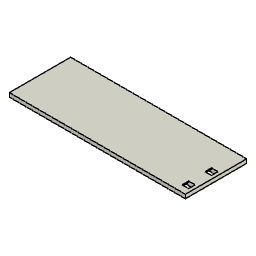
sorted_smarties_top_panel (Autodesk Fusion 360 design; units mm, degrees)
Autodesk Fusion 360 part; units mm, degrees
sketch "Sorted Smarties Top" plane through (0, 0, 0) normal (0, 0, 1) x (1, 0, 0)
  line L0 (0, 0) -> (-270, 0)
  line L1 (-270, 0) -> (-270, 94)
  line L2 (-270, 94) -> (0, 94)
  line L3 (0, 94) -> (0, 0)
  dimension "d2" = 270
  dimension "d3" = 94
  constraint horizontal L0
  constraint vertical L1
  constraint horizontal L2
  constraint vertical L3
  constraint coincident L0.start L3.end
  measures "d2" distance of L0.start L0.end
  measures "d3" distance of L0.start L2.end
extrude "Extrude1" add sketch "Sorted Smarties Top" along normal blind 6
sketch "Sketch2" plane through (0, 0, 0) normal (0, 0, -1) x (1, 0, 0)
  line L0 (-270, -94) -> (0, -94)
  line L1 (0, -94) -> (0, 0)
  line L2 (0, 0) -> (-270, 0)
  line L3 (-270, 0) -> (-270, -94)
  line L4 (-5, -10) -> (-265, -10)
  line L5 (-265, -10) -> (-265, -20)
  line L6 (-265, -20) -> (-5, -20)
  line L7 (-5, -20) -> (-5, -10)
  line L8 (-5, -45) -> (-265, -45)
  line L9 (-265, -45) -> (-265, -55)
  line L10 (-265, -55) -> (-5, -55)
  line L11 (-5, -55) -> (-5, -45)
  dimension "d6" = 10
  dimension "d7" = 10
  dimension "d8" = 10
  dimension "d9" = 25
  dimension "d10" = 5
  dimension "d11" = 5
  dimension "d12" = 5
  dimension "d13" = 5
  constraint horizontal L4
  constraint vertical L5
  constraint horizontal L6
  constraint vertical L7
  constraint horizontal L8
  constraint vertical L9
  constraint horizontal L10
  constraint vertical L11
  measures "d6" distance of L2 L4
  measures "d7" distance of L4.start L6.end
  measures "d8" distance of L8.start L10.end
  measures "d9" distance of L6 L8
  measures "d10" distance of L3 L5
  measures "d11" distance of L1 L7
  measures "d12" distance of L1 L11
  measures "d13" distance of L3 L9
extrude "Extrude2" cut sketch "Sketch2" against normal blind 4 contours L4 L5 L6 L7 | L8 L9 L10 L11
sketch "Sketch3" plane through (0, 0, 4) normal (0, 0, -1) x (1, 0, 0)
  line L0 (-5, -20) -> (-5, -10)
  line L1 (-5, -10) -> (-265, -10)
  line L2 (-265, -10) -> (-265, -20)
  line L3 (-265, -20) -> (-5, -20)
  line L4 (-5, -10) -> (-15, -10)
  line L5 (-15, -10) -> (-15, -20)
  line L6 (-15, -20) -> (-5, -20)
  line L7 (-5, -20) -> (-5, -10)
  line L8 (-5, -45) -> (-15, -45)
  line L9 (-15, -45) -> (-15, -55)
  line L10 (-15, -55) -> (-5, -55)
  line L11 (-5, -55) -> (-5, -45)
  constraint horizontal L4
  constraint vertical L5
  constraint horizontal L6
  constraint vertical L7
  constraint coincident L3 L5.end
  constraint coincident L0.end L1.start
  constraint horizontal L8
  constraint vertical L9
  constraint horizontal L10
  constraint vertical L11
extrude "Extrude3" cut sketch "Sketch3" against normal blind 2 contours L0 L1 L3 L4 L5 L6 L7 | L8 L9 L10 L11
equation "MDFThickness = 6 mm" comment "Thickness of the MDF board."
equation "d3 = 100 mm - MDFThickness"
equation "d4 = MDFThickness"
named bodies: "Sorted Smarties Top Panel"
